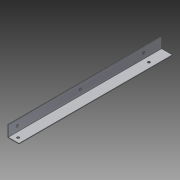
# Autodesk Inventor part: Hopper Bracing Right Leg P13
Saved by Autodesk Inventor 2014 SP1 (Build 180222100, 222)
## iProperties
Created: 2013-12-16
Part Number: Hopper Bracing Right Leg P13
Material: Aluminum 6061
Document SubType Name: Modeling
Designer: Moses
Mass: 14.2772 g
Surface Area: 137.092 cm^2
Volume: 5.26834 cm^3
Density: 2.71 g/cm^3
Appearance: Aluminum - Flat
Author: Moses
Autodesk Inventor part; units mm, degrees
ref_plane "YZ Plane" through (0, 0, 0) normal (1, 0, 0) x (0, 1, 0)
ref_plane "XZ Plane" through (0, 0, 0) normal (0, 1, 0) x (-1, 0, 0)
ref_plane "XY Plane" through (0, 0, 0) normal (0, 0, 1) x (1, 0, 0)
sketch "Sketch1" plane through (0, 0, 0) normal (0, 0, 1) x (1, 0, 0)
  line L0 (0, 0) -> (0, 15.875)
  line L1 (0, 15.875) -> (0.7937, 15.875)
  line L2 (0.7937, 15.875) -> (0.7938, 0.7937)
  line L3 (0.7938, 0.7937) -> (15.875, 0.7937)
  line L4 (15.875, 0.7937) -> (15.875, 0)
  line L5 (15.875, 0) -> (0, 0)
  dimension "d0" = 15.875
  dimension "d1" = 0.7937
  constraints: 12 end point, 3 horizontal, 3 vertical, 2 perpendicular
  measures "d0" distance of L0.start L0.end
  measures "d1" distance of L0.end L1.end
extrude "Extrusion1" add sketch "Sketch1" along normal blind 215.9
sketch "Sketch2" plane through (0.7938, 0.7937, 0) normal (0, 1, 0) x (1, 0, 0)
  line L0 (0, 0) -> (15.0812, 0) projected
  line L1 (15.0812, -215.9) -> (0, -215.9) projected
  line L2 (7.5406, 0) -> (7.5406, -215.9) construction
  circle A0 centre (7.5406, -25.4) radius 1.7145
  circle A1 centre (7.5406, -209.55) radius 1.7145
  point P0 (-0.7938, 0)
  dimension "d4" = 25.4
  dimension "d5" = 3.429
  dimension "d6" = 215.9
  dimension "d28" = 6.35
  constraints: 2 centre point, 2 end point, 2 midpoint, 2 point on line, 1 equal radius
  measures "d4" distance from line of L0 A0.centre
  measures "d5" diameter of A0
  measures "d6" distance of L0.end L1.start
  measures "d28" distance of A1.centre L2.end
sketch "Sketch3" plane through (0.7938, 0.7937, 0) normal (1, 0, 0) x (0, 0, -1)
  line L0 (0, 15.0812) -> (0, 0) projected
  line L1 (-215.9, 0) -> (-215.9, 15.0812) projected
  line L2 (-215.9, 7.5406) -> (0, 7.5406) construction
  circle A0 centre (-25.4, 7.5406) radius 1.7145
  circle A1 centre (-114.3, 7.5406) radius 1.7145
  circle A2 centre (-203.2, 7.5406) radius 1.7145
  point P0 (0, -0.7937)
  dimension "d14" = 3.429
  dimension "d15" = 25.4
  dimension "d16" = 215.9
  dimension "d19" = 88.9
  constraints: 3 centre point, 2 end point, 2 midpoint, 1 horizontal, 1 point on line, 4 other
  measures "d14" diameter of A0
  measures "d15" distance of L2.end A0.centre
  measures "d16" distance of L0.start L1.end
  measures "d19" distance of A0.centre A1.centre
extrude "Extrusion2" cut sketch "Sketch2" against normal through all
extrude "Extrusion3" cut sketch "Sketch3" against normal through all
body "Solid1"
